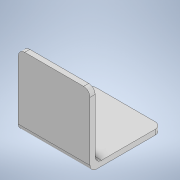
# Autodesk Inventor part: sideplatemount
Saved by Autodesk Inventor 2020.1 (Build 241239000, 239)
## iProperties
Created: 2019-12-09
Part Number: sideplatemount
Material: Generic
Document SubType Name: Modeling
Designer: tbloo
Density: 1 g/cm^3
Appearance: Default
Author: tbloo
Autodesk Inventor part; units mm, degrees
ref_plane "YZ Plane" through (0, 0, 0) normal (1, 0, 0) x (0, 1, 0)
ref_plane "XZ Plane" through (0, 0, 0) normal (0, 1, 0) x (-1, 0, 0)
ref_plane "XY Plane" through (0, 0, 0) normal (0, 0, 1) x (1, 0, 0)
sketch "Sketch1" plane through (0, 0, 0) normal (1, 0, 0) x (0, 1, 0)
  line L0 (0, 0) -> (28, 0)
  line L1 (28, 0) -> (28, -2)
  line L2 (0, -2) -> (0, 0)
  line L3 (0, 0) -> (2, 0)
  line L4 (2, -28) -> (0, -28)
  line L5 (0, -28) -> (0, 0)
  line L6 (28, -2) -> (2, -2)
  line L7 (2, -2) -> (2, -28)
  dimension "d0" = 28
  dimension "d1" = 2
  dimension "d2" = 2
  dimension "d3" = 28
  constraints: 16 end point, 3 perpendicular, 2 horizontal, 2 parallel
  measures "d0" distance of L1.end L2.start
  measures "d1" distance of L0.end L1.end
  measures "d2" distance of L4.start L4.end
  measures "d3" distance of L3.end L4.start
extrude "Extrusion1" add sketch "Sketch1" along normal blind 28
fillet "Fillet1" radius 2.5 6 edges at (28, 28, -1) (0, 28, -1) (28, 1, -28) (0, 1, -28) (14, 2, -2) (14, 0, 0)
body "Solid1"
